Autodesk Fusion 360 part; units mm, degrees
(part 2 of 2)
  line L358 (-4.2706, -29.2818) -> (-4.2706, -42.2818)
  line L359 (-17.7706, -28.7818) -> (-4.7706, -28.7818)
  arc A358 (84.6232, 9.3182) -> (84.1232, 8.8182) centre (84.6232, 8.8182) ccw
  line L360 (60.8107, 14.3682) -> (73.8107, 14.3682)
  line L361 (-63.0143, 52.4682) -> (-50.0143, 52.4682)
  arc A359 (92.8607, 14.3682) -> (93.3607, 14.8682) centre (92.8607, 14.8682) ccw
  line L362 (89.3857, -28.7818) -> (102.3857, -28.7818)
  line L363 (-64.2706, -44.7818) -> (-58.2706, -44.7818)
  line L364 (-146.7143, 73.4682) -> (167.0357, 73.4682)
  line L365 (167.0357, 73.4682) -> (167.0357, -49.7818)
  line L366 (167.0357, -49.7818) -> (-146.7143, -49.7818)
  line L367 (-146.7143, -49.7818) -> (-146.7143, 73.4682)
  dimension "d3" = 366.214
  dimension "d4" = 150.212
  dimension "d5" = 16.317
  dimension "d6" = 21.381
  dimension "d7" = 15
  dimension "d8" = 15
  dimension "d9" = 25
  dimension "d10" = 32
  dimension "d11" = 2.9
  dimension "d12" = 5.5
  dimension "d13" = 5.5
  dimension "d14" = 2.9
  dimension "d15" = 5.5
  dimension "d16" = 5.5
  dimension "d17" = 2.9
  dimension "d18" = 5.5
  dimension "d19" = 5.5
  dimension "d20" = 2.9
  dimension "d21" = 5.5
  dimension "d22" = 5.5
  dimension "d23" = 7
  dimension "d24" = 7
  dimension "d25" = 7
  dimension "d26" = 7
  constraint horizontal L14
  constraint vertical L341
  constraint horizontal L13
  constraint vertical L198
  constraint horizontal L225
  constraint vertical L15
  constraint horizontal L246
  constraint vertical L17
  constraint horizontal L364
  constraint vertical L365
  constraint horizontal L366
  constraint vertical L367
  measures "d3" distance of L198 L341
  measures "d4" distance of L13 L14
  measures "d5" distance of L157 L198
  measures "d6" distance of L13 L174
  measures "d7" distance of L225 L246
  measures "d8" distance of L15 L17
  measures "d9" distance of L15 L341
  measures "d10" distance of L13 L246
  measures "d11" diameter of A102
  measures "d12" distance of A102.centre L341
  measures "d13" distance of A102.centre L13
  measures "d14" diameter of A13
  measures "d15" distance of A13.centre L341
  measures "d16" distance of A13.centre L14
  measures "d17" diameter of A25
  measures "d18" distance of A25.centre L13
  measures "d19" distance of A25.centre L198
  measures "d20" diameter of A65
  measures "d21" distance of A65.centre L14
  measures "d22" distance of A65.centre L198
  measures "d23" distance of L108 L366
  measures "d24" distance of L322 L365
  measures "d25" distance of L3 L364
  measures "d26" distance of L57 L367
extrude "Extrude1" add sketch "Sketch1" along normal blind 12 contours L13 L14 L198 L341
fillet "Fillet1" radius 7 4 edges at (212.5639, -64.1628, 6) (212.5639, 86.0492, 6) (-153.6501, 86.0492, 6) (-153.6501, -64.1628, 6)
fillet "Fillet2" radius 4 8 edges at (210.5137, -62.1126, 12) (212.5639, 10.9432, 12) (210.5137, 83.9989, 12) (29.4569, 86.0492, 12) (-151.5998, 83.9989, 12) (-153.6501, 10.9432, 12) (-151.5998, -62.1126, 12) (29.4569, -64.1628, 12)
fillet "Fillet3" radius 2 4 edges at (10.1607, 73.4682, 12) (-146.7143, 11.8432, 12) (167.0357, 11.8432, 12) (10.1607, -49.7818, 12)
fillet "Fillet4" radius 2 4 edges at (180.0639, -17.1628, 12) (172.5639, -24.6628, 12) (180.0639, -32.1628, 12) (187.5639, -24.6628, 12)
